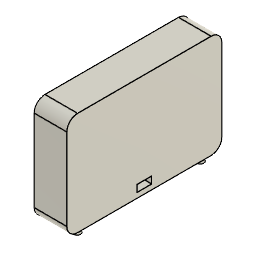
GridNote (Autodesk Fusion 360 design; units mm, degrees)
part number: 2026-03-08-10-30-58-446
Autodesk Fusion 360 part; units mm, degrees
note: some values were not read from the file. Set by a fixed rule: which sketch regions a step uses.
sketch "Sketch1" plane through (0, 0, 0) normal (0, 0, 1) x (1, 0, 0)
sketch "Sketch2" plane through (0, 0, 0) normal (1, 0, 0) x (0, 1, 0)
  line L0 (4, 11) -> (159, 11)
  line L1 (171.5, -1.5) -> (171.5, -96.5)
  line L2 (159, -109) -> (4, -109)
  line L3 (-8.5, -96.5) -> (-8.5, -1.5)
  line L4 (0, 0) -> (163, 0)
  line L5 (163, 0) -> (163, -98)
  line L6 (163, -98) -> (0, -98)
  line L7 (0, -98) -> (0, 0)
  arc A0 (4, 11) -> (-8.5, -1.5) centre (4, -1.5) ccw
  arc A1 (171.5, -1.5) -> (159, 11) centre (159, -1.5) ccw
  arc A2 (159, -109) -> (171.5, -96.5) centre (159, -96.5) ccw
  arc A3 (-8.5, -96.5) -> (4, -109) centre (4, -96.5) ccw
  point P0 (-8.5, 11)
  point P1 (171.5, 11)
  point P2 (-8.5, -109)
  dimension "d1" = 120
  dimension "d2" = 180
  dimension "d3" = 98
  dimension "d4" = 163
  dimension "d5" = 11
  dimension "d6" = 8.5
  dimension "d13" = 12.5
  constraint horizontal L0
  constraint vertical L1
  constraint horizontal L2
  constraint vertical L3
  constraint horizontal L4
  constraint vertical L5
  constraint horizontal L6
  constraint vertical L7
  constraint coincident L4.start L7.end
  constraint coincident P0 L0
  constraint coincident P0 L3
  constraint tangent L0 A0
  constraint tangent L3 A0
  constraint coincident P1 L0
  constraint coincident P1 L1
  constraint tangent L0 A1
  constraint tangent L1 A1
  constraint equal A0 A1
  constraint tangent L1 A2
  constraint tangent L2 A2
  constraint equal A0 A2
  constraint coincident P2 L2
  constraint coincident P2 L3
  constraint tangent L2 A3
  constraint tangent L3 A3
  constraint equal A0 A3
  measures "d1" distance of P0 P2
  measures "d2" distance of P0 P1
  measures "d3" distance of L4.start L6.end
  measures "d4" distance of L4.start L4.end
  measures "d5" distance of L0 L4
  measures "d6" distance of L3 L7
  measures "d13" radius of A0
extrude "Extrude1" add sketch "Sketch2" along normal blind 2
extrude "Extrude2" add 1 faces at (0, 107.3333, 3.6667) along direction (-1, 0, 0) blind 33
sketch "Sketch3" plane through (2, 0, 0) normal (1, 0, 0) x (0, 1, 0)
  line L0 (163, -98) -> (0, -98)
  line L1 (0, -98) -> (0, 0)
  line L2 (0, 0) -> (163, 0)
  line L3 (163, 0) -> (163, -98)
  line L4 (4, -109) -> (159, -109)
  line L5 (171.5, -96.5) -> (171.5, -1.5)
  line L6 (159, 11) -> (4, 11)
  line L7 (-8.5, -1.5) -> (-8.5, -96.5)
  line L8 (-8.5, -1.5) -> (159, -1.5)
  line L9 (159, -1.5) -> (159, -109)
  line L10 (159, -109) -> (-8.5, -109)
  line L11 (-8.5, -109) -> (-8.5, -1.5)
  arc A0 (4, 11) -> (-8.5, -1.5) centre (4, -1.5) ccw
  arc A1 (-8.5, -96.5) -> (4, -109) centre (4, -96.5) ccw
  arc A2 (159, -109) -> (171.5, -96.5) centre (159, -96.5) ccw
  arc A3 (171.5, -1.5) -> (159, 11) centre (159, -1.5) ccw
  constraint horizontal L8
  constraint vertical L9
  constraint horizontal L10
  constraint vertical L11
  constraint coincident L4.end L9.end
  constraint coincident L7.start L8.start
sketch "Sketch4" plane through (2, 0, 0) normal (1, 0, 0) x (0, 1, 0)
  line L0 (163, -98) -> (0, -98)
  line L1 (0, -98) -> (0, 0)
  line L2 (0, 0) -> (163, 0)
  line L3 (163, 0) -> (163, -98)
  arc A0 (4, 11) -> (-8.5, -1.5) centre (4, -1.5) ccw
  line L4 (-8.5, -1.5) -> (-8.5, -96.5)
  arc A1 (-8.5, -96.5) -> (4, -109) centre (4, -96.5) ccw
  line L5 (4, -109) -> (159, -109)
  arc A2 (159, -109) -> (171.5, -96.5) centre (159, -96.5) ccw
  line L6 (171.5, -96.5) -> (171.5, -1.5)
  arc A3 (171.5, -1.5) -> (159, 11) centre (159, -1.5) ccw
  line L7 (159, 11) -> (4, 11)
  line L8 (0, 0) -> (163, 0)
  line L9 (163, 0) -> (163, -98)
  line L10 (163, -98) -> (0, -98)
  line L11 (0, -98) -> (0, 0)
  line L12 (-10, 10) -> (-94.6711, 10)
  line L13 (-94.6711, 10) -> (-94.6711, 7.3388)
  line L14 (-94.6711, 7.3388) -> (-10, 7.3388)
  line L15 (-10, 7.3388) -> (-10, 10)
  constraint horizontal L8
  constraint vertical L9
  constraint horizontal L10
  constraint vertical L11
  constraint coincident L0.start L3.end
  constraint coincident L1.end L2.start
  constraint horizontal L12
  constraint vertical L13
  constraint horizontal L14
  constraint vertical L15
extrude "Extrude4" add sketch "Sketch4" along normal blind 3 contours L0 L1 L2 L3 L8 L9 L10 L11 | A0 L4 A1 L5 A2 L6 A3 L7
sketch "Sketch5" plane through (0, 0, -109) normal (0, 0, -1) x (1, 0, 0)
  line L0 (-33, -159) -> (5, -159)
  line L1 (5, -159) -> (5, -4)
  line L2 (5, -4) -> (-33, -4)
  line L3 (-33, -4) -> (-33, -159)
  circle A0 centre (-26.5, -10) radius 4
  circle A1 centre (-1.5, -10) radius 4
  circle A2 centre (-26.5, -153) radius 4
  circle A3 centre (-1.5, -153) radius 4
  dimension "d16" = 8
  dimension "d17" = 8
  dimension "d18" = 8
  dimension "d19" = 8
  dimension "d20" = 6
  dimension "d21" = 6
  dimension "d22" = 6
  dimension "d23" = 6
  dimension "d24" = 6.5
  dimension "d25" = 6.5
  dimension "d26" = 6.5
  dimension "d27" = 6.5
  measures "d16" diameter of A0
  measures "d17" diameter of A1
  measures "d18" diameter of A2
  measures "d19" diameter of A3
  measures "d20" distance of L2 A0.centre
  measures "d21" distance of L2 A1.centre
  measures "d22" distance of L0 A2.centre
  measures "d23" distance of L0 A3.centre
  measures "d24" distance of L1 A3.centre
  measures "d25" distance of L3 A2.centre
  measures "d26" distance of L1 A1.centre
  measures "d27" distance of L3 A0.centre
extrude "Extrude5" add sketch "Sketch5" along normal blind 6 contours A0 | A1 | A2 | A3
sketch "Sketch6" plane through (5, 0, 0) normal (1, 0, 0) x (0, 1, 0)
  line L0 (159, 11) -> (4, 11)
  arc A0 (4, 11) -> (-8.5, -1.5) centre (4, -1.5) ccw
  line L1 (-8.5, -1.5) -> (-8.5, -96.5)
  arc A1 (-8.5, -96.5) -> (4, -109) centre (4, -96.5) ccw
  line L2 (4, -109) -> (159, -109)
  arc A2 (159, -109) -> (171.5, -96.5) centre (159, -96.5) ccw
  line L3 (171.5, -96.5) -> (171.5, -1.5)
  arc A3 (171.5, -1.5) -> (159, 11) centre (159, -1.5) ccw
  line L4 (73, -95) -> (82, -95)
  line L5 (82, -103) -> (73, -103)
  line L6 (73, -95) -> (90, -95)
  line L7 (90, -95) -> (90, -103)
  line L8 (90, -103) -> (73, -103)
  line L9 (73, -103) -> (73, -95)
  constraint horizontal L4
  constraint horizontal L5
  constraint horizontal L6
  constraint vertical L7
  constraint horizontal L8
  constraint vertical L9
extrude "Extrude7" cut sketch "Sketch6" against normal blind 10 contours L4 L5 L6 L7 L8 L9
